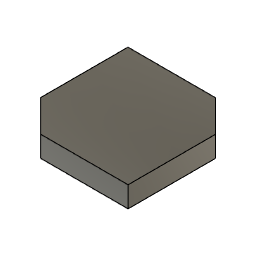
EMRG (Autodesk Fusion 360 design; units mm, degrees)
Autodesk Fusion 360 part; units mm, degrees
sketch "Sketch1" plane through (0, 0, 0) normal (0, 0, 1) x (1, 0, 0)
  line L0 (0, 0) -> (5.725, 0) construction
  line L1 (5.725, 0) -> (5.725, -5.717) construction
  line L2 (5.725, -5.717) -> (0, -5.717) construction
  line L3 (0, -5.717) -> (0, 0) construction
  line L4 (0, 0) -> (4.208, 0)
  line L5 (0, 0) -> (0, -4.192)
  line L6 (5.725, -5.717) -> (1.525, -5.717)
  line L7 (5.725, -5.717) -> (5.725, -1.517)
  line L8 (0, -4.192) -> (1.525, -5.717)
  line L9 (4.208, 0) -> (5.725, -1.517)
  dimension "d1" = 5.725
  dimension "d2" = 5.717
  dimension "d3" = 4.208
  dimension "d4" = 4.192
  dimension "d5" = 4.2
  dimension "d6" = 4.2
  constraint horizontal L0
  constraint vertical L1
  constraint horizontal L2
  constraint vertical L3
  constraint coincident L0.start L3.end
  constraint perpendicular L3 L4
  constraint parallel L3 L5
  constraint perpendicular L1 L6
  constraint perpendicular L6 L7
  measures "d1" distance of L0.start L0.end
  measures "d2" distance of L0.start L2.end
  measures "d3" distance of L0.start L4.end
  measures "d4" distance of L0.start L5.end
  measures "d5" distance of L1.end L6.end
  measures "d6" distance of L1.end L7.end
extrude "Extrude1" add sketch "Sketch1" along normal blind 1
scale "Scale1" factor 1.25 about (4.208, 0, 0) bodies 1
